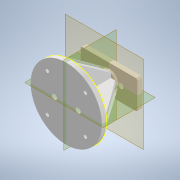
# Autodesk Inventor part: gripper extension
Saved by Autodesk Inventor 2021 (Build 250183000, 183)
## iProperties
Created: 2023-03-19
Part Number: gripper extension
Material: Generic
Document SubType Name: Modeling
Designer: mahmo
Density: 1 g/cm^3
Appearance: Default
Author: mahmo
Autodesk Inventor part; units mm, degrees
ref_plane "YZ Plane" through (0, 0, 0) normal (1, 0, 0) x (0, 1, 0)
ref_plane "XZ Plane" through (0, 0, 0) normal (0, 1, 0) x (-1, 0, 0)
ref_plane "XY Plane" through (0, 0, 0) normal (0, 0, 1) x (1, 0, 0)
sketch "Sketch1" plane through (0, 0, 0) normal (0, 0, 1) x (1, 0, 0)
  circle A0 centre (11, 0) radius 3.5 projected
  circle A1 centre (36, 0) radius 3.5 projected
  arc A2 (0, 2.7354) -> (0.3, 2.6) centre (0.3, 3) ccw projected
  line L0 (0.3, 2.6) -> (1, 2.6) projected
  arc A3 (1, 2.6) -> (1.2, 2.8) centre (1, 2.8) ccw projected
  line L1 (1.2, 2.8) -> (1.2, 3.05) projected
  arc A4 (1.4, 3.25) -> (1.2, 3.05) centre (1.4, 3.05) ccw projected
  line L2 (1.4, 3.25) -> (4, 3.25) projected
  arc A5 (4.4, 2.85) -> (4, 3.25) centre (4, 2.85) ccw projected
  line L3 (4.4, 2.85) -> (4.4, -2.85) projected
  arc A6 (4, -3.25) -> (4.4, -2.85) centre (4, -2.85) ccw projected
  line L4 (4, -3.25) -> (1.4, -3.25) projected
  arc A7 (1.2, -3.05) -> (1.4, -3.25) centre (1.4, -3.05) ccw projected
  line L5 (1.2, -3.05) -> (1.2, -2.8) projected
  arc A8 (1.2, -2.8) -> (1, -2.6) centre (1, -2.8) ccw projected
  line L6 (1, -2.6) -> (0.3, -2.6) projected
  arc A9 (0.3, -2.6) -> (0, -2.7354) centre (0.3, -3) ccw projected
  line L7 (0, -2.7354) -> (0, -11) projected
  line L8 (47, -11) -> (0, -11) projected
  line L9 (47, -11) -> (47, -2.7354) projected
  arc A10 (47, -2.7354) -> (46.7, -2.6) centre (46.7, -3) ccw projected
  line L10 (46.7, -2.6) -> (46, -2.6) projected
  arc A11 (46, -2.6) -> (45.8, -2.8) centre (46, -2.8) ccw projected
  line L11 (45.8, -2.8) -> (45.8, -3.05) projected
  arc A12 (45.6, -3.25) -> (45.8, -3.05) centre (45.6, -3.05) ccw projected
  line L12 (45.6, -3.25) -> (43, -3.25) projected
  arc A13 (42.6, -2.85) -> (43, -3.25) centre (43, -2.85) ccw projected
  line L13 (42.6, -2.85) -> (42.6, 2.85) projected
  arc A14 (43, 3.25) -> (42.6, 2.85) centre (43, 2.85) ccw projected
  line L14 (43, 3.25) -> (45.6, 3.25) projected
  arc A15 (45.8, 3.05) -> (45.6, 3.25) centre (45.6, 3.05) ccw projected
  line L15 (45.8, 3.05) -> (45.8, 2.8) projected
  arc A16 (45.8, 2.8) -> (46, 2.6) centre (46, 2.8) ccw projected
  line L16 (46, 2.6) -> (46.7, 2.6) projected
  arc A17 (46.7, 2.6) -> (47, 2.7354) centre (46.7, 3) ccw projected
  line L17 (47, 2.7354) -> (47, 11) projected
  line L18 (0, 11) -> (47, 11) projected
  line L19 (0, 11) -> (0, 2.7354) projected
  line L20 (23.5, -11) -> (23.5, 11) construction
  line L21 (0, 0) -> (47, 0) construction
  line L22 (53.5, -15) -> (-6.5, -15)
  line L23 (-6.5, -15) -> (-6.5, 15)
  line L24 (-6.5, 15) -> (53.5, 15)
  line L25 (53.5, 15) -> (53.5, -15)
  line L26 (53.5, -15) -> (-6.5, 15) construction
  line L27 (-6.5, -15) -> (53.5, 15) construction
  point P0 (23.5, 0)
  dimension "d0" = 60
  dimension "d1" = 30
  constraints: 16 end point, 5 midpoint, 2 horizontal, 2 parallel, 1 perpendicular
  measures "d0" distance of L23.end L24.end
  measures "d1" distance of L22.end L23.end
extrude "Extrusion1" add sketch "Sketch1" against normal blind 2 contours L22 L23 L24 L25
sketch "Sketch2" plane through (0, 0, 0) normal (0, 0, 1) x (1, 0, 0)
  line L0 (-6.5, -15) -> (-6.5, 15) projected
  line L1 (53.5, -15) -> (-6.5, -15)
  line L2 (-6.5, -15) -> (-6.5, 15)
  line L3 (-6.5, 15) -> (53.5, 15)
  line L4 (53.5, 15) -> (53.5, -15)
  circle A0 centre (11, 0) radius 3.5 projected
  circle A1 centre (36, 0) radius 3.5 projected
  arc A2 (0, 2.7354) -> (0.3, 2.6) centre (0.3, 3) ccw projected
  line L5 (0.3, 2.6) -> (1, 2.6) projected
  arc A3 (1, 2.6) -> (1.2, 2.8) centre (1, 2.8) ccw projected
  line L6 (1.2, 2.8) -> (1.2, 3.05) projected
  arc A4 (1.4, 3.25) -> (1.2, 3.05) centre (1.4, 3.05) ccw projected
  line L7 (1.4, 3.25) -> (4, 3.25) projected
  arc A5 (4.4, 2.85) -> (4, 3.25) centre (4, 2.85) ccw projected
  line L8 (4.4, 2.85) -> (4.4, -2.85) projected
  arc A6 (4, -3.25) -> (4.4, -2.85) centre (4, -2.85) ccw projected
  line L9 (4, -3.25) -> (1.4, -3.25) projected
  arc A7 (1.2, -3.05) -> (1.4, -3.25) centre (1.4, -3.05) ccw projected
  line L10 (1.2, -3.05) -> (1.2, -2.8) projected
  arc A8 (1.2, -2.8) -> (1, -2.6) centre (1, -2.8) ccw projected
  line L11 (1, -2.6) -> (0.3, -2.6) projected
  arc A9 (0.3, -2.6) -> (0, -2.7354) centre (0.3, -3) ccw projected
  line L12 (0, -2.7354) -> (0, -11) projected
  line L13 (47, -11) -> (0, -11) projected
  line L14 (47, -11) -> (47, -2.7354) projected
  arc A10 (47, -2.7354) -> (46.7, -2.6) centre (46.7, -3) ccw projected
  line L15 (46.7, -2.6) -> (46, -2.6) projected
  arc A11 (46, -2.6) -> (45.8, -2.8) centre (46, -2.8) ccw projected
  line L16 (45.8, -2.8) -> (45.8, -3.05) projected
  arc A12 (45.6, -3.25) -> (45.8, -3.05) centre (45.6, -3.05) ccw projected
  line L17 (45.6, -3.25) -> (43, -3.25) projected
  arc A13 (42.6, -2.85) -> (43, -3.25) centre (43, -2.85) ccw projected
  line L18 (42.6, -2.85) -> (42.6, 2.85) projected
  arc A14 (43, 3.25) -> (42.6, 2.85) centre (43, 2.85) ccw projected
  line L19 (43, 3.25) -> (45.6, 3.25) projected
  arc A15 (45.8, 3.05) -> (45.6, 3.25) centre (45.6, 3.05) ccw projected
  line L20 (45.8, 3.05) -> (45.8, 2.8) projected
  arc A16 (45.8, 2.8) -> (46, 2.6) centre (46, 2.8) ccw projected
  line L21 (46, 2.6) -> (46.7, 2.6) projected
  arc A17 (46.7, 2.6) -> (47, 2.7354) centre (46.7, 3) ccw projected
  line L22 (47, 2.7354) -> (47, 11) projected
  line L23 (0, 11) -> (47, 11) projected
  line L24 (0, 11) -> (0, 2.7354) projected
  point P0 (0, 0)
  constraints: 8 end point, 2 parallel, 1 horizontal, 1 perpendicular
extrude "Extrusion2" add sketch "Sketch2" along normal blind 3 contours L0 L3 L4 L1 | L24 L23 L22 A17 L21 A16 L20 A15 L19 A14 L18 A13 L17 A12 L16 A11 L15 A10 L14 L13 L12 A9 L11 A8 L10 A7 L9 A6 L8 A5 L7 A4 L6 A3 L5 A2
sketch "Sketch3" plane through (0, 0, 3) normal (0, 0, 1) x (1, 0, 0)
  circle A0 centre (36, 0) radius 2.65 projected
  circle A1 centre (11, 0) radius 2.65 projected
  circle A2 centre (11, 0) radius 3.5 projected
  circle A3 centre (36, 0) radius 3.5 projected
  point P0 (0, 0)
ref_plane "Work Plane1" through (0, -11, 0) normal (0, 0, 1) x (1, 0, 0)
extrude "Extrusion3" add sketch "Sketch3" against normal up to surface (3 mm away)
sketch "Sketch4" plane through (0, 0, 0) normal (0, 0, -1) x (-1, 0, 0)
  point P0 (0, 0)
sketch "Sketch5" plane through (0, 0, 0) normal (0, 0, -1) x (-1, 0, 0)
  circle A0 centre (-36, 0) radius 3.5 projected
  circle A1 centre (-11, 0) radius 3.5 projected
  circle A2 centre (-11, 0) radius 2.65 projected
  circle A3 centre (-36, 0) radius 2.65 projected
  point P0 (0, 0)
extrude "Extrusion4" cut sketch "Sketch5" against normal blind 1.4 contours A0 | A1 | A2 | A3
ref_plane "Work Plane3" through (0, 0, 43) normal (0, 0, 1) x (1, 0, 0)
sketch "Sketch6" plane through (0, 0, 43) normal (0, 0, 1) x (1, 0, 0)
  circle A0 centre (11, 0) radius 2.65 construction
  circle A1 centre (36, 0) radius 2.65 construction
  line L0 (53.5, -15) -> (53.5, 15) construction
  line L1 (53.5, 15) -> (-6.5, 15) construction
  line L2 (-6.5, 15) -> (-6.5, -15) construction
  line L3 (-6.5, -15) -> (53.5, -15) construction
  line L4 (-6.5, -15) -> (-6.5, 15) construction
  line L5 (-6.5, 0) -> (53.5, 0) construction
  line L6 (53.5, -15) -> (-6.5, -15) construction
  line L7 (23.5, -15) -> (23.5, 15) construction
  line L8 (-6.5, 15) -> (53.5, 15) construction
  circle A2 centre (23.5, 0) radius 37.5
  point P0 (0, 0)
  dimension "d12" = 75
  constraints: 5 midpoint, 4 end point, 1 centre point
  measures "d12" diameter of A2
extrude "Extrusion5" add sketch "Sketch6" along normal blind 5
sketch "Sketch7" plane through (0, 0, 3) normal (0, 0, 1) x (1, 0, 0)
  circle A0 centre (23.5, 0) radius 9.85
  constraints: 1 centre point, 1 coincident
sketch "Sketch8" plane through (23.5, 0, 43) normal (0, 0, -1) x (-1, 0, 0)
  circle A0 centre (0, 0) radius 37.5 projected
  point P0 (23.5, 0)
loft "Loft1" add profiles "Sketch7" section 2 edges at (-14, 0, 43)
sketch "Sketch10" plane through (0, 0, 3) normal (0, 0, 1) x (1, 0, 0)
  line L0 (-6.5, -15) -> (53.5, -15) construction
  line L1 (23.5, -15) -> (23.5, 15) construction
  line L2 (-6.5, 15) -> (53.5, 15) construction
  line L3 (53.5, -15) -> (53.5, 15) construction
  line L4 (53.5, 0) -> (-6.5, 0) construction
  line L5 (-6.5, 15) -> (-6.5, -15) construction
  line L6 (53.5, -4) -> (-6.5, -4)
  line L7 (-6.5, -4) -> (-6.5, 4)
  line L8 (-6.5, 4) -> (53.5, 4)
  line L9 (53.5, 4) -> (53.5, -4)
  line L10 (53.5, -4) -> (-6.5, 4) construction
  line L11 (-6.5, -4) -> (53.5, 4) construction
  line L12 (-14, 4) -> (61, 4)
  line L13 (61, 4) -> (61, -4)
  line L14 (61, -4) -> (-14, -4)
  line L15 (-14, -4) -> (-14, 4)
  arc A0 (33.35, 0) -> (13.65, 0) centre (23.5, 0) ccw projected
  line L16 (-14, 4) -> (61, -4) construction
  line L17 (61, 4) -> (-14, -4) construction
  point P0 (0, 0)
  dimension "d22" = 8
  dimension "d28" = 75
  constraints: 28 end point, 9 midpoint, 4 parallel, 2 horizontal, 2 perpendicular, 1 point on line
  measures "d22" distance of L6.end L7.end
  measures "d28" distance of L13.end L14.end
extrude "Extrusion7" cut sketch "Sketch10" along normal blind 38 contours L6 L7 L8 L9 | L9 L12 L13 L14 | L14 L15 L12 L7
sketch "Sketch11" plane through (0, 0, 3) normal (0, 0, 1) x (1, 0, 0)
  line L0 (19.5, -37.5) -> (27.5, -37.5)
  line L1 (27.5, -37.5) -> (27.5, 37.5)
  line L2 (27.5, 37.5) -> (19.5, 37.5)
  line L3 (19.5, 37.5) -> (19.5, -37.5)
  line L4 (19.5, -37.5) -> (27.5, 37.5) construction
  line L5 (27.5, -37.5) -> (19.5, 37.5) construction
  point P0 (0, 0)
  point P1 (23.5, 0)
  dimension "d29" = 8
  dimension "d30" = 75
  constraints: 12 end point, 2 midpoint, 2 parallel, 1 horizontal, 1 perpendicular
  measures "d29" distance of L2.end L1.end
  measures "d30" distance of L1.end L0.end
extrude "Extrusion8" cut sketch "Sketch11" along normal blind 38
sketch "Sketch9" plane through (23.5, 0, 48) normal (0, 0, 1) x (1, 0, 0)
  circle A0 centre (-12.5, 0) radius 2.65 projected
  circle A1 centre (12.5, 0) radius 2.65 projected
  point P0 (-23.5, 0)
extrude "Extrusion6" cut sketch "Sketch9" against normal through all
sketch "Sketch12" plane through (0, 0, 3) normal (0, 0, 1) x (1, 0, 0)
  point P0 (0, 0)
ref_plane "Work Plane4" through (23.5, 0, 8) normal (0, 0, 1) x (1, 0, 0)
sketch "Sketch13" plane through (23.5, 0, 8) normal (0, 0, 1) x (1, 0, 0)
  circle A0 centre (0, 0) radius 37.5 projected
  circle A1 centre (12.5, 0) radius 2.65 projected
  circle A2 centre (-12.5, 0) radius 2.65 projected
  line L0 (-35.8953, -4) -> (-4, -4) projected
  arc A3 (-35.8953, 4) -> (-35.8953, -4) centre (0, 0) ccw
  line L1 (-4, 4) -> (-35.8953, 4) projected
  line L2 (-4, 35.8953) -> (-4, 4) projected
  arc A4 (4, 35.8953) -> (-4, 35.8953) centre (0, 0) ccw
  line L3 (4, 4) -> (4, 35.8953) projected
  line L4 (35.8953, 4) -> (4, 4) projected
  line L5 (4, -4) -> (35.8953, -4) projected
  line L6 (4, -35.8953) -> (4, -4) projected
  arc A5 (-4, -35.8953) -> (4, -35.8953) centre (0, 0) ccw
  line L7 (-4, -4) -> (-4, -35.8953) projected
  line L8 (35.8953, -4) -> (37.2861, -4)
  line L9 (35.8953, 4) -> (37.2861, 4)
  line L10 (-35.8953, 4) -> (-37.2861, 4)
  line L11 (-35.8953, -4) -> (-37.2861, -4)
  line L12 (-4, 35.8953) -> (-4, 37.2861)
  arc A6 (4, 35.8953) -> (-4, 35.8953) centre (0, 0) ccw projected
  line L13 (4, 35.8953) -> (4, 37.2861)
  circle A7 centre (0, 0) radius 37.5 projected
  arc A8 (-4, -35.8953) -> (4, -35.8953) centre (0, 0) ccw projected
  line L14 (-4, -35.8953) -> (-4, -37.2861)
  line L15 (4, -35.8953) -> (4, -37.2861)
  line L16 (-4, -37.2861) -> (-7, -37.2861) construction
  line L17 (-7, -37.2861) -> (-7, -33.2861) construction
  line L18 (-7, -33.2861) -> (-4, -33.2861) construction
  line L19 (-4, -33.2861) -> (-4, -37.2861) construction
  line L20 (-37.2861, -4) -> (-33.2861, -4) construction
  line L21 (-33.2861, -4) -> (-33.2861, -7) construction
  line L22 (-33.2861, -7) -> (-37.2861, -7) construction
  line L23 (-37.2861, -7) -> (-37.2861, -4) construction
  line L24 (-36.8409, -7) -> (52.5452, -7)
  line L25 (-7, -36.8409) -> (-7, 43.9269)
  point P0 (-23.5, 0)
  point P1 (-7, -36.8409)
  point P2 (-7, -7)
  dimension "d32" = 3
  dimension "d33" = 4
  dimension "d34" = 4
  dimension "d35" = 3
  constraints: 36 end point, 8 point on line, 7 centre point, 6 parallel, 6 point on circle, 3 horizontal, 3 perpendicular, 12 other
  measures "d32" distance of L17.end L18.end
  measures "d33" distance of L16.end L17.end
  measures "d34" distance of L21.end L22.end
  measures "d35" distance of L20.end L21.end
extrude "Extrusion9" cut sketch "Sketch13" along normal blind 34.5 contours A0 L24 L25
ref_plane "Work Plane5" through (14.4988, 0, 3) normal (0, -1, 0) x (1, 0, 0)
ref_plane "Work Plane6" through (23.5, -9.0012, 3) normal (-1, 0, 0) x (0, 0, 1)
mirror "Mirror1" about plane through (14.4988, 0, 3) normal (0, -1, 0) of "Extrusion9"
mirror "Mirror2" about plane through (23.5, -9.0012, 3) normal (-1, 0, 0) of "Extrusion9", "Mirror1"
sketch "Sketch14" plane through (0, 0, 3) normal (0, 0, 1) x (1, 0, 0)
  point P0 (0, 0)
sketch "Sketch15" plane through (0, 0, 3) normal (0, 0, 1) x (1, 0, 0)
  arc A0 (14.4988, -4) -> (19.5, -9.0012) centre (23.5, 0) ccw projected
  circle A1 centre (23.5, 0) radius 9.5
  point P0 (0, 0)
  point P1 (14.4988, -4)
  dimension "d40" = 19
  constraints: 1 centre point, 1 coincident
  measures "d40" diameter of A1
extrude "Extrusion10" add sketch "Sketch15" along normal blind 40
fillet "Fillet1" radius 2 4 edges at (53.5, -15, 0.5) (-6.5, -15, 0.5) (53.5, 15, 0.5) (-6.5, 15, 0.5)
sketch "Sketch18" plane through (59.989, -7, 42.5) normal (0, 0, -1) x (-1, 0, 0)
  circle A0 centre (16.489, -13) radius 1.75 projected
  circle A1 centre (56.489, -13) radius 1.75 projected
  circle A2 centre (56.489, 27) radius 1.75 projected
  circle A3 centre (16.489, 27) radius 1.75 projected
  point P0 (59.989, 7)
extrude "Extrusion12" cut sketch "Sketch18" against normal blind 10
body "Solid1"
